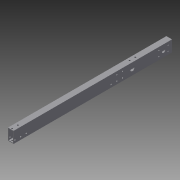
# Autodesk Inventor part: 2x1
Saved by Autodesk Inventor 2015 SP1 (Build 190203100, 203)
## iProperties
Created: 2015-01-14
Part Number: 2x1
Material: Generic
Document SubType Name: Modeling
Designer: 215152
Density: 1 g/cm^3
Appearance: Default
Author: 215152
Autodesk Inventor part; units mm, degrees
ref_plane "YZ Plane" through (0, 0, 0) normal (1, 0, 0) x (0, 1, 0)
ref_plane "XZ Plane" through (0, 0, 0) normal (0, 1, 0) x (-1, 0, 0)
ref_plane "XY Plane" through (0, 0, 0) normal (0, 0, 1) x (1, 0, 0)
sketch "Sketch1" plane through (0, 0, 0) normal (0, 0, 1) x (1, 0, 0)
  line L0 (0, 0) -> (25.4, 0)
  line L1 (25.4, 0) -> (25.4, 50.8)
  line L2 (25.4, 50.8) -> (0, 50.8)
  line L3 (0, 50.8) -> (0, 0)
  line L4 (3.175, 3.175) -> (22.225, 3.175)
  line L5 (22.225, 3.175) -> (22.225, 47.625)
  line L6 (22.225, 47.625) -> (3.175, 47.625)
  line L7 (3.175, 47.625) -> (3.175, 3.175)
  dimension "d0" = 25.4
  dimension "d1" = 50.8
  dimension "d2" = 19.05
  dimension "d3" = 44.45
  dimension "d4" = 3.175
  dimension "d5" = 3.175
  constraints: 16 end point, 4 parallel, 2 horizontal, 2 perpendicular
  measures "d0" distance of L2.end L1.end
  measures "d1" distance of L1.end L0.end
  measures "d2" distance of L6.end L5.end
  measures "d3" distance of L5.end L4.end
  measures "d4" distance between parallel lines of L0 L4
  measures "d5" distance between parallel lines of L3 L7
extrude "Extrusion1" add sketch "Sketch1" along normal blind 711.2
sketch "Sketch9" plane through (0, 50.8, 0) normal (0, 1, 0) x (1, 0, 0)
  line L0 (25.4, 0) -> (0, 0) projected
  line L1 (0, 0) -> (0, -711.2) projected
  line L2 (25.4, -711.2) -> (0, -711.2) projected
  line L3 (25.4, 0) -> (25.4, -711.2) projected
  point P0 (12.7, -704.85)
  point P1 (12.7, -679.45)
  point P2 (12.7, -203.2)
  point P3 (12.7, -177.8)
  dimension "d75" = 6.35
  dimension "d76" = 12.7
  dimension "d77" = 12.7
  dimension "d78" = 31.75
  dimension "d79" = 12.7
  dimension "d80" = 12.7
  dimension "d81" = 508
  dimension "d82" = 533.4
  measures "d75" distance from line of point (12.7, -704.85) L2
  measures "d76" distance from line of L1 point (12.7, -704.85)
  measures "d77" distance from line of L1 point (12.7, -679.45)
  measures "d78" distance from line of point (12.7, -679.45) L2
  measures "d79" distance from line of L3 point (12.7, -203.2)
  measures "d80" distance from line of L3 point (12.7, -177.8)
  measures "d81" distance from line of L2 point (12.7, -203.2)
  measures "d82" distance from line of L2 point (12.7, -177.8)
hole "Hole6" at (12.7, 50.8, 704.85) at (12.7, 50.8, 679.45) at (12.7, 50.8, 203.2) at (12.7, 50.8, 177.8) direction (0, -1, 0) diameter 6.35 end through all
sketch "Sketch10" plane through (0, 0, 0) normal (-1, 0, 0) x (0, 0, 1)
  line L0 (0, 50.8) -> (0, 0) projected
  line L1 (0, 0) -> (711.2, 0) projected
  line L2 (711.2, 50.8) -> (711.2, 0) projected
  line L3 (0, 50.8) -> (711.2, 50.8) projected
  point P0 (704.85, 12.7)
  point P1 (679.45, 12.7)
  point P2 (273.05, 12.7)
  point P3 (247.65, 12.7)
  point P4 (222.25, 12.7)
  point P5 (654.05, 12.7)
  dimension "d90" = 6.35
  dimension "d91" = 12.7
  dimension "d92" = 12.7
  dimension "d93" = 31.75
  dimension "d94" = 12.7
  dimension "d95" = 12.7
  dimension "d96" = 438.15
  dimension "d97" = 463.55
  dimension "d130" = 12.7
  dimension "d131" = 488.95
  dimension "d132" = 12.7
  dimension "d133" = 57.15
  measures "d90" distance from line of L2 point (704.85, 12.7)
  measures "d91" distance from line of L1 point (704.85, 12.7)
  measures "d92" distance from line of L1 point (679.45, 12.7)
  measures "d93" distance from line of L2 point (679.45, 12.7)
  measures "d94" distance from line of L1 point (273.05, 12.7)
  measures "d95" distance from line of L1 point (247.65, 12.7)
  measures "d96" distance from line of L2 point (273.05, 12.7)
  measures "d97" distance from line of L2 point (247.65, 12.7)
  measures "d130" distance from line of L1 point (222.25, 12.7)
  measures "d131" distance from line of L2 point (222.25, 12.7)
  measures "d132" distance from line of L1 point (654.05, 12.7)
  measures "d133" distance from line of L2 point (654.05, 12.7)
sketch "Sketch11" plane through (0, 0, 0) normal (-1, 0, 0) x (0, 0, 1)
  line L0 (0, 50.8) -> (0, 0) projected
  line L1 (0, 0) -> (711.2, 0) projected
  line L2 (711.2, 50.8) -> (711.2, 0) projected
  line L3 (0, 50.8) -> (711.2, 50.8) projected
  point P0 (190.5, 25.4)
  dimension "d105" = 25.4
  dimension "d129" = 520.7
  measures "d105" distance from line of L1 point (190.5, 25.4)
  measures "d129" distance from line of L2 point (190.5, 25.4)
hole "Hole8" at (0, 25.4, 190.5) direction (1, 0, 0) diameter 19.05 end through all
hole "Hole10" at (0, 12.7, 704.85) at (0, 12.7, 679.45) at (0, 12.7, 273.05) at (0, 12.7, 247.65) at (0, 12.7, 222.25) at (0, 12.7, 654.05) direction (1, 0, 0) diameter 6.35 end through all
sketch "Sketch13" plane through (25.4, 0, 0) normal (1, 0, 0) x (0, 0, -1)
  circle A0 centre (-222.25, 12.7) radius 3.175 projected
  circle A1 centre (-273.05, 12.7) radius 3.175 projected
  circle A2 centre (-704.85, 12.7) radius 3.175 projected
  circle A3 centre (-679.45, 12.7) radius 3.175 projected
  circle A4 centre (-247.65, 12.7) radius 3.175 projected
  circle A5 centre (-654.05, 12.7) radius 3.175 projected
  circle A6 centre (-190.5, 25.4) radius 9.525 projected
  line L0 (0, 0) -> (0, 50.8) projected
  line L1 (0, 50.8) -> (-711.2, 50.8) projected
  line L2 (-711.2, 0) -> (-711.2, 50.8) projected
  line L3 (0, 0) -> (-711.2, 0) projected
  point P0 (-247.65, 38.1)
  point P1 (-222.25, 38.1)
  dimension "d141" = 12.7
  dimension "d142" = 12.7
  dimension "d143" = 463.55
  dimension "d144" = 488.95
  measures "d141" distance from line of L1 point (-247.65, 38.1)
  measures "d142" distance from line of L1 point (-222.25, 38.1)
  measures "d143" distance from line of L2 point (-247.65, 38.1)
  measures "d144" distance from line of point (-222.25, 38.1) L2
hole "Hole11" at (25.4, 38.1, 247.65) at (25.4, 38.1, 222.25) direction (-1, 0, 0) diameter 6.35 end through all
sketch "Sketch14" plane through (25.4, 0, 0) normal (1, 0, 0) x (0, 0, -1)
  circle A0 centre (-247.65, 38.1) radius 3.175 projected
  circle A1 centre (-222.25, 38.1) radius 3.175 projected
  circle A2 centre (-222.25, 12.7) radius 3.175 projected
  circle A3 centre (-273.05, 12.7) radius 3.175 projected
  circle A4 centre (-704.85, 12.7) radius 3.175 projected
  circle A5 centre (-679.45, 12.7) radius 3.175 projected
  circle A6 centre (-247.65, 12.7) radius 3.175 projected
  circle A7 centre (-654.05, 12.7) radius 3.175 projected
  circle A8 centre (-190.5, 25.4) radius 9.525 projected
  line L0 (0, 0) -> (0, 50.8) projected
  line L1 (0, 50.8) -> (-711.2, 50.8) projected
  line L2 (-711.2, 0) -> (-711.2, 50.8) projected
  line L3 (0, 0) -> (-711.2, 0) projected
  line L4 (-38.1, 25.4) -> (-17.4778, 37.3062) construction
  line L5 (-38.1, 25.4) -> (-14.2875, 25.4) construction
  line L6 (-38.1, 25.4) -> (-17.4778, 13.4938) construction
  line L7 (-38.1, 25.4) -> (-14.2875, 25.4) construction
  line L8 (-38.1, 25.4) -> (-58.7222, 37.3063) construction
  line L9 (-38.1, 25.4) -> (-14.2875, 25.4) construction
  line L10 (-38.1, 25.4) -> (-58.7222, 13.4938) construction
  line L11 (-38.1, 25.4) -> (-14.2875, 25.4) construction
  circle A9 centre (-38.1, 25.4) radius 7.9375
  circle A10 centre (-58.7222, 37.3063) radius 2.54
  circle A11 centre (-58.7222, 13.4938) radius 2.54
  circle A12 centre (-17.4778, 13.4938) radius 2.54
  circle A13 centre (-17.4778, 37.3062) radius 2.54
  dimension "d152" = 38.1
  dimension "d153" = 25.4
  dimension "d154" = 23.8125
  dimension "d155" = 30
  dimension "d156" = 23.8125
  dimension "d157" = 30
  dimension "d158" = 23.8125
  dimension "d159" = 150
  dimension "d160" = 23.8125
  dimension "d161" = 150
  dimension "d162" = 15.875
  dimension "d163" = 5.08
  dimension "d164" = 5.08
  dimension "d165" = 5.08
  dimension "d166" = 5.08
  constraints: 16 end point, 9 coincident, 5 centre point, 4 equal length, 4 horizontal
  measures "d152" distance from line of L0 L4.start
  measures "d153" distance from line of L3 L4.start
  measures "d154" distance of L4.start L4.end
  measures "d155" angle of L5 L4
  measures "d156" distance of L4.start L6.end
  measures "d157" angle of L6 L7
  measures "d158" distance of L4.start L8.end
  measures "d159" angle of L9 L8
  measures "d160" distance of L4.start L10.end
  measures "d161" angle of L10 L11
  measures "d162" diameter of A9
  measures "d163" diameter of A10
  measures "d164" diameter of A11
  measures "d165" diameter of A12
  measures "d166" diameter of A13
extrude "Extrusion4" cut sketch "Sketch14" against normal blind 25.4 contours A9 | A10 | A11 | A12 | A13
body "Solid1"
